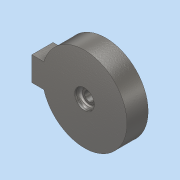
# Autodesk Inventor part: 编码器模型
Saved by Autodesk Inventor 2019 (Build 230136000, 136)
## iProperties
Created: 2020-10-24
Part Number: 编码器模型
Material: Generic
Document SubType Name: Modeling
Designer: Wang Hua
Density: 1 g/cm^3
Appearance: 镀锌
Author: Wang Hua
Autodesk Inventor part; units mm, degrees
ref_plane "YZ Plane" through (0, 0, 0) normal (1, 0, 0) x (0, 1, 0)
ref_plane "XZ Plane" through (0, 0, 0) normal (0, 1, 0) x (-1, 0, 0)
ref_plane "XY Plane" through (0, 0, 0) normal (0, 0, 1) x (1, 0, 0)
sketch "草图1" plane through (0, 0, 0) normal (0, 0, 1) x (1, 0, 0)
  arc A0 (-13.4198, -3.9887) -> (-13.4198, 3.9887) centre (0, 0) ccw
  line L0 (-13.4198, -3.9887) -> (-17.3861, -3.9887)
  line L1 (-17.3861, -3.9887) -> (-17.3861, 3.9887)
  line L2 (-17.3861, 3.9887) -> (-13.4198, 3.9887)
  line L3 (-9.2259, -3.9887) -> (-17.3861, 3.9887) construction
  line L4 (-17.3861, -3.9887) -> (-9.2259, 3.9887) construction
  circle A1 centre (0, 0) radius 1.6
  point P0 (-13.306, 0)
  dimension "d0" = 14
  dimension "d1" = 3.2
  constraints: 10 end point, 2 centre point, 2 coincident, 2 midpoint, 2 point on circle, 1 horizontal, 1 parallel, 1 perpendicular
  measures "d0" radius of A0
  measures "d1" diameter of A1
extrude "拉伸1" add sketch "草图1" along normal blind 7
sketch "草图2" plane through (0, 0, 0) normal (0, 0, -1) x (-1, 0, 0)
  circle A0 centre (0, 0) radius 10
  dimension "d4" = 20
  constraints: 1 centre point, 1 coincident
  measures "d4" diameter of A0
extrude "拉伸2" cut sketch "草图2" against normal blind 3
sketch "草图3" plane through (0, 0, 7) normal (0, 0, 1) x (1, 0, 0)
  circle A0 centre (0, 0) radius 3.25
  dimension "d7" = 6.5
  constraints: 1 centre point, 1 coincident
  measures "d7" diameter of A0
extrude "拉伸3" cut sketch "草图3" against normal blind 1.6
fillet "圆角1" radius 1 1 edges at (-3.25, 0, 5.4)
